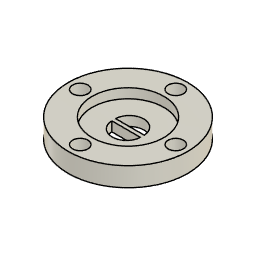
Gear Potentionmeter Joint (Autodesk Fusion 360 design; units mm, degrees)
Autodesk Fusion 360 part; units mm, degrees
sketch "スケッチ1" plane through (0, 0, 0) normal (0, 0, 1) x (1, 0, 0)
  circle A0 centre (0, 0) radius 7.5
  circle A1 centre (0, 0) radius 10
  line L0 (0, 0) -> (10, 0)
  line L1 (0, 0) -> (-10, 0)
  line L2 (0, 0) -> (0, -10)
  circle A2 centre (-10, 0) radius 1.6
  circle A3 centre (10, 0) radius 1.6
  circle A4 centre (0, -10) radius 1.6
  circle A5 centre (0, 0) radius 12.5
  arc A6 (-3, -0.3) -> (3, -0.3) centre (0, -0.3) ccw
  line L3 (3, 0.3) -> (-3, 0.3)
  line L4 (-3, -0.3) -> (3, -0.3)
  arc A7 (3, 0.3) -> (-3, 0.3) centre (0, 0.3) ccw
  line L5 (0, 0) -> (0, 10)
  circle A8 centre (0, 10) radius 1.6
  dimension "d1" = 15
  dimension "d2" = 20
  dimension "d3" = 3.2
  dimension "d4" = 3.2
  dimension "d5" = 3.2
  dimension "d6" = 25
  dimension "d11" = 3.2
  constraint coincident A0.centre A1.centre
  constraint concentric A0 A1
  constraint coincident A1 L0.end
  constraint horizontal L0
  constraint coincident A1 L1.end
  constraint parallel L0 L1
  constraint coincident A1 L2.end
  constraint perpendicular L1 L2
  constraint coincident L1.end A2.centre
  constraint coincident L0.end A3.centre
  constraint coincident L2.end A4.centre
  constraint perpendicular L3 L5
  constraint coincident L5.end A8.centre
  measures "d1" diameter of A0
  measures "d2" diameter of A1
  measures "d3" diameter of A2
  measures "d4" diameter of A3
  measures "d5" diameter of A4
  measures "d6" diameter of A5
  measures "d11" diameter of A8
extrude "押し出し1" add sketch "スケッチ1" along normal blind 2 contours A0 L0 L3 A7 L5 | A0 A1 L0 L2 A3 A4 | A0 L0 L2 A6 L4 | A0 A1 L0 A3 L5 A8 | A0 L1 L3 A7 L5 | A0 A1 L1 A2 L5 A8 | A0 A1 L1 L2 A2 A4 | A0 L1 L2 A6 L4 | A5
extrude "押し出し2" add sketch "スケッチ1" against normal blind 2 contours A0 A1 L0 L2 A3 A4 | A0 A1 L0 A3 L5 A8 | A0 A1 L1 A2 L5 A8 | A0 A1 L1 L2 A2 A4 | A5
move_body "移動1" bodies 1 to x (1, 0, 0) y (0, -1, 0) z (0, 0, -1) at (0, 0, 0)
sketch "スケッチ2" plane through (0, 0, 0) normal (0, 0, 1) x (-1, 0, 0)
  circle A0 centre (0, 0) radius 7.5
  arc A1 (3, 0.3) -> (-3, 0.3) centre (0, 0.3) ccw
  line L0 (3, 0.3) -> (-3, 0.3)
  arc A2 (-3, -0.3) -> (3, -0.3) centre (0, -0.3) ccw
  line L1 (-3, -0.3) -> (3, -0.3)
  line L2 (3, -0.3) -> (3, 0.3)
  line L3 (-3, -0.3) -> (-3, 0.3)
  line L4 (-3, 0.4) -> (3, 0.4)
  line L5 (3, 0.4) -> (3, -0.4)
  line L6 (3, -0.4) -> (-3, -0.4)
  line L7 (-3, -0.4) -> (-3, 0.4)
  line L8 (-3, 0.4) -> (3, -0.4) construction
  line L9 (3, 0.4) -> (-3, -0.4) construction
  dimension "d13" = 6
  dimension "d14" = 0.8
  constraint coincident A2.end L1.end
  constraint coincident A1.start L0.start
  constraint coincident A2.start L1.start
  constraint coincident A1.end L0.end
  constraint horizontal L4
  constraint perpendicular L4 L5
  constraint parallel L4 L6
  constraint parallel L5 L7
  constraint coincident L8 A0.centre
  constraint coincident L9 A0.centre
  constraint coincident A0.centre origin
  measures "d13" distance of L5.end L6.end
  measures "d14" distance of L4.end L5.end
extrude "押し出し3" add sketch "スケッチ2" against normal blind 2 contours A1 L0 L4 L5 L7 | A2 L1 L5 L6 L7
extrude "押し出し4" add 1 faces at (6.8696, 3.9313, -2) along direction (0, 0, -1) blind 1
extrude "押し出し5" cut 1 faces at (6.8696, 3.9313, -3) along direction (0, 0, 1) blind 1
